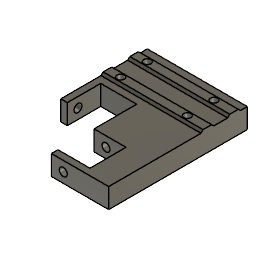
Fixed Roller Bracket A (Autodesk Fusion 360 design; units mm, degrees)
part number: 2026-05-27-15-50-34-677
Autodesk Fusion 360 part; units mm, degrees
note: some values were not read from the file. Set by a fixed rule: which sketch regions a step uses.
sketch "Sketch1" plane through (0, 0, 0) normal (0, 0, 1) x (1, 0, 0)
  line L0 (-25, -15) -> (-25, 50)
  line L1 (-25, 50) -> (50, 50)
  line L2 (50, 50) -> (50, -54)
  line L3 (-20, -15) -> (-20, 10)
  line L4 (-20, 10) -> (7, 10)
  line L5 (7, -22) -> (7, 10)
  line L6 (-19, -7) -> (6, -7)
  line L7 (-25, -15) -> (-20, -15)
  line L8 (7, -22) -> (31, -22)
  line L9 (16, -23) -> (16, -48)
  line L10 (-19, -20) -> (6, -20) construction
  line L11 (-19, 6) -> (6, 6) construction
  line L12 (29, -23) -> (29, -48) construction
  line L13 (31, -22) -> (31, -49)
  line L14 (7, -49) -> (31, -49)
  line L15 (7, -54) -> (50, -54)
  line L16 (7, -49) -> (7, -54)
  circle A0 centre (-15, 20) radius 2.7
  circle A1 centre (35, 20) radius 2.7
  circle A2 centre (-15, 40) radius 2.7
  circle A3 centre (35, 40) radius 2.7
  line L17 (3, -23) -> (3, -48) construction
  line L18 (3, -23) -> (29, -23) construction
  line L19 (3, -48) -> (29, -48) construction
  line L20 (-19, 6) -> (-19, -20) construction
  line L21 (6, 6) -> (6, -20) construction
  dimension "d10" = 5.4
  dimension "d13" = 50
  dimension "d14" = 20
  dimension "d35" = 25
  dimension "d36" = 1
  dimension "d37" = 25
  dimension "d38" = 1
  dimension "d39" = 65
  constraint parallel L0 L2
  constraint perpendicular L3 L7
  constraint perpendicular L5 L8
  constraint perpendicular L8 L9
  constraint perpendicular L15 L16
  constraint perpendicular L12 L18
  constraint perpendicular L12 L19
  constraint perpendicular L10 L20
  constraint perpendicular L10 L21
  constraint coincident L6.start L20
  constraint coincident L6.end L21
  constraint coincident L9.start L18
  constraint coincident L9.end L19
  measures "d10" diameter of A0
  measures "d35" distance of L9.start L9.end
  measures "d36" distance of L8 L9.start
  measures "d37" distance of L6.start L6.end
  measures "d38" distance of L5 L6.end
  measures "d39" distance of L1 L7
extrude "Extrude1" add sketch "Sketch1" along normal blind 15
sketch "Sketch2" plane through (-25, 0, 0) normal (-1, 0, 0) x (0, -1, 0)
  line L0 (-50, 0) -> (15, 0)
  line L1 (15, 0) -> (15, 15)
  line L2 (15, 15) -> (-50, 15)
  line L3 (-50, 15) -> (-50, 0)
  circle A0 centre (7, 7.5) radius 3
  point P0 (5, 0)
  dimension "d17" = 6
  measures "d17" diameter of A0
sketch "Sketch4" plane through (0, -54, 0) normal (0, -1, 0) x (1, 0, 0)
  line L0 (7, 0) -> (50, 0)
  line L1 (50, 0) -> (50, 15)
  line L2 (50, 15) -> (7, 15)
  line L3 (7, 15) -> (7, 0)
  circle A0 centre (16, 7.5) radius 3
  point P0 (16, 0)
  dimension "d18" = 6
  measures "d18" diameter of A0
extrude "Extrude2" cut sketch "Sketch2" against normal blind 40 contours A0
extrude "Extrude3" cut sketch "Sketch4" against normal blind 40 contours A0
sketch "Sketch5" plane through (-25, 0, 0) normal (-1, 0, 0) x (0, -1, 0)
  line L0 (-35.2, 15) -> (-44.8, 15)
  line L1 (-36.8, 16.6) -> (-43.2, 16.6)
  line L2 (-15.2, 15) -> (-24.8, 15)
  line L3 (-16.8, 16.6) -> (-23.2, 16.6)
  line L4 (-16.8, 16.6) -> (-15.2, 15)
  line L5 (-16.8, 16.6) -> (-14.5373, 16.6) construction
  line L6 (-23.2, 16.6) -> (-24.8, 15)
  line L7 (-23.2, 16.6) -> (-20.9373, 16.6) construction
  line L8 (-36.8, 16.6) -> (-35.2, 15)
  line L9 (-36.8, 16.6) -> (-34.5373, 16.6) construction
  line L10 (-43.2, 16.6) -> (-44.8, 15)
  dimension "d40" = 45
  dimension "d41" = 135
  dimension "d42" = 45
  constraint horizontal L5
  constraint horizontal L7
  constraint horizontal L9
  constraint perpendicular L8 L10
  measures "d40" angle of L4 L5
  measures "d41" angle of L6 L7
  measures "d42" angle of L8 L9
extrude "Extrude4" add sketch "Sketch5" against normal blind 75
sketch "Sketch6" plane through (0, 0, 15) normal (0, 0, 1) x (-1, 0, 0)
  line L0 (25, -15.2) -> (25, 15)
  line L1 (25, 15) -> (20, 15)
  line L2 (20, 15) -> (20, -10)
  line L3 (20, -10) -> (-7, -10)
  line L4 (-7, -10) -> (-7, 22)
  line L5 (-7, 22) -> (-31, 22)
  line L6 (-31, 22) -> (-31, 49)
  line L7 (-31, 49) -> (-7, 49)
  line L8 (-7, 49) -> (-7, 54)
  line L9 (-7, 54) -> (-50, 54)
  line L10 (-50, 54) -> (-50, -15.2)
  circle A0 centre (15, -40) radius 2.7
  circle A1 centre (15, -20) radius 2.7
  circle A2 centre (-35, -20) radius 2.7
  circle A3 centre (-35, -40) radius 2.7
  line L11 (-50, -15.2) -> (25, -15.2)
  point P0 (15, -40)
  point P1 (15, -20)
  point P2 (-35, -20)
  point P3 (-35, -40)
  constraint coincident P0 A0.centre
  constraint coincident P1 A1.centre
  constraint coincident P2 A2.centre
  constraint coincident P3 A3.centre
extrude "Extrude5" cut sketch "Sketch6" along normal blind 1.8 contours A0 | A1 | A2 | A3
sketch "Sketch3" plane through (0, 0, 0) normal (0, 0, 1) x (1, 0, 0)
  point P0 (16, -69.9704)
  point P1 (16, -69.9704)
named bodies: "Fixed Roller Bracket A"
